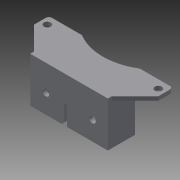
# Autodesk Inventor part: support
Saved by Autodesk Inventor 2015 (Build 190159000, 159)
## iProperties
Created: 2014-08-15
Part Number: support
Material: Generic
Document SubType Name: Modeling
Designer: Christo
Density: 1 g/cm^3
Appearance: Default
Author: Christo
Autodesk Inventor part; units mm, degrees
ref_plane "YZ Plane" through (0, 0, 0) normal (1, 0, 0) x (0, 1, 0)
ref_plane "XZ Plane" through (0, 0, 0) normal (0, 1, 0) x (-1, 0, 0)
ref_plane "XY Plane" through (0, 0, 0) normal (0, 0, 1) x (1, 0, 0)
sketch "Sketch1" plane through (0, 0, 0) normal (0, 0, 1) x (1, 0, 0)
  line L0 (-40, -40) -> (-40, 40) construction
  line L1 (40, -40) -> (-40, -40) construction
  line L2 (40, 40) -> (40, -40) construction
  circle A0 centre (35.75, -35.75) radius 2.25 construction
  circle A1 centre (-35.75, -35.75) radius 2.25 construction
  circle A2 centre (0, 0) radius 35.75 construction
  line L3 (-40, -40) -> (-25, -55)
  line L4 (-40, -40) -> (-18.7868, -40) construction
  line L5 (-25, -55) -> (25, -55)
  line L6 (25, -55) -> (40, -40)
  line L7 (-40, -40) -> (-40, -30.4857)
  line L8 (40, -40) -> (40, -30.4857)
  circle A3 centre (0, 0) radius 38.75 construction
  circle A4 centre (35.75, -35.75) radius 2.25
  circle A5 centre (-35.75, -35.75) radius 2.25
  line L9 (-40, -30.4857) -> (-18.673, -30.4857)
  line L10 (40, -30.4857) -> (18.673, -30.4857)
  arc A6 (-18.673, -30.4857) -> (18.673, -30.4857) centre (0, 0) ccw
extrude "Extrusion3" add sketch "Sketch1" along normal blind 2.5
sketch "Sketch5" plane through (-25, -55, 0) normal (0, -1, 0) x (1, 0, 0)
  line L0 (50, 2.5) -> (0, 2.5)
  line L1 (0, 2.5) -> (0, -26.5)
  line L2 (0, -26.5) -> (50, -26.5)
  line L3 (50, -26.5) -> (50, 2.5)
  point P0 (25, 0)
  dimension "d22" = 29
  constraints: 8 end point, 2 parallel, 1 horizontal, 1 perpendicular
  measures "d22" distance of L0.end L1.end
extrude "Extrusion5" add sketch "Sketch5" along normal blind 2.5
sketch "Sketch6" plane through (-25, -55, 0) normal (0, 1, 0) x (1, 0, 0)
  line L0 (40, 14) -> (10, 14)
  point P0 (25, 0)
  point P1 (25, 0)
  point P2 (25, 14)
  dimension "d25" = 30
  dimension "d52" = 14
  constraints: 2 end point, 1 horizontal, 1 midpoint, 1 vertical alignment
  measures "d25" distance of L0.start L0.end
  measures "d52" distance from line of L0 point (25, 0)
hole "Hole2" at (15, -55, -14) at (-15, -55, -14) direction (0, -1, 0) diameter 4.5 end through all
fillet "Fillet2" radius 2 2 edges at (40, -30.4857, 1.25) (-40, -30.4857, 1.25)
sketch "Sketch8" plane through (0, 0, 0) normal (0, 0, -1) x (-1, 0, 0)
  line L0 (-40, -40) -> (40, -40) construction
  line L1 (-40, 40) -> (-40, -40) construction
  line L2 (40, 40) -> (-40, 40) construction
  line L3 (40, -40) -> (40, 40) construction
  circle A0 centre (35.75, -35.75) radius 2.25 construction
  circle A1 centre (35.75, 35.75) radius 2.25 construction
  circle A2 centre (-35.75, 35.75) radius 2.25 construction
  circle A3 centre (-35.75, -35.75) radius 2.25 construction
  circle A4 centre (0, 0) radius 38.75 construction
  line L4 (-25, -55) -> (-22.5, -55)
  line L5 (-22.5, -55) -> (-22.5, -40)
  line L6 (-22.5, -40) -> (-25, -40)
  line L7 (-25, -40) -> (-25, -55)
  line L8 (25, -55) -> (22.5, -55)
  line L9 (22.5, -55) -> (22.5, -40)
  line L10 (22.5, -40) -> (25, -40)
  line L11 (25, -40) -> (25, -55)
  line L12 (25, -55) -> (-25, -55) projected
  line L13 (1.25, -55) -> (-1.25, -55)
  line L14 (-1.25, -55) -> (-1.25, -40)
  line L15 (-1.25, -40) -> (1.25, -40)
  line L16 (1.25, -40) -> (1.25, -55)
  point P0 (0, -40)
  dimension "d39" = 2.5
  dimension "d40" = 2.5
  dimension "d41" = 2.5
  constraints: 24 end point, 6 parallel, 3 horizontal, 3 perpendicular, 3 point on line, 2 midpoint, 1 vertical alignment
  measures "d39" distance of L6.end L5.end
  measures "d40" distance of L9.end L10.end
  measures "d41" distance of L14.end L15.end
extrude "Extrusion7" add sketch "Sketch8" along normal up to surface (26.5 mm away)
sketch "Sketch9" plane through (-25, -57.5, 0) normal (0, -1, 0) x (1, 0, 0)
  line L0 (23.75, 0) -> (23.75, -26.5) construction
  line L1 (23.75, 0) -> (23.75, -26.5) construction
  circle A0 centre (40, -14) radius 2.25 construction
  circle A1 centre (10, -14) radius 2.25 construction
  line L2 (40, -14) -> (10, -14) construction
  line L3 (23.75, -26.5) -> (21.75, -26.5)
  line L4 (21.75, -26.5) -> (21.75, -14)
  line L5 (21.75, -14) -> (23.75, -14)
  line L6 (23.75, -14) -> (23.75, -26.5)
  point P0 (25, 0)
  dimension "d45" = 2
  constraints: 10 end point, 2 horizontal, 2 parallel, 1 perpendicular, 1 point on line
  measures "d45" distance of L1.end L3.end
extrude "Extrusion8" cut sketch "Sketch9" against normal through all
fillet "Fillet3" radius 1 2 edges at (-1.25, -56.25, -14) (-3.25, -56.25, -14)
fillet "Fillet4" radius 2 1 edges at (-3.25, -56.25, -26.5)
equation "\"d23\" = ep"
equation "\"d39\" = ep"
equation "\"d40\" = ep"
equation "\"d41\" = ep"
equation "\"d42\" = ep"
equation "\"d46\" = ep"
equation "\"d44\" = A1"
equation "\"ep\" = 2.5"
equation "\"A1\" = 45deg"
body "Solid1"
body "Solid2"
